Autodesk Inventor part; units mm, degrees
(part 2 of 5)
  line L843 (-13.4881, 9.0142) -> (-14.9433, 10.4694)
  line L844 (-14.9433, 10.4694) -> (-17.5891, 16.2902)
  line L845 (-17.5891, 16.2902) -> (-17.8537, 18.4068)
  line L846 (-17.8537, 18.4068) -> (-18.2506, 18.6714)
  line L847 (-18.2506, 18.6714) -> (-18.6474, 18.4068)
  line L848 (-18.6474, 18.4068) -> (-20.2349, 15.4964)
  line L849 (-20.2349, 15.4964) -> (-21.5972, 16.8588)
  line L850 (-21.5972, 16.8588) -> (-22.7485, 18.4068)
  line L851 (-22.7485, 18.4068) -> (-22.1661, 18.9123)
  line L852 (-22.1661, 18.9123) -> (-21.4256, 19.2006)
  line L853 (-21.4256, 19.2006) -> (-21.2443, 19.7141)
  line L854 (-21.2443, 19.7141) -> (-21.272, 20.1719)
  line L855 (-21.272, 20.1719) -> (-21.5088, 20.574)
  line L856 (-21.5088, 20.574) -> (-21.9547, 20.9204)
  line L857 (-21.9547, 20.9204) -> (-23.5422, 21.185)
  line L858 (-23.5422, 21.185) -> (-24.1862, 22.076)
  line L859 (-24.1862, 22.076) -> (-25.1297, 22.6402)
  line L860 (-25.1297, 22.6402) -> (-25.5266, 22.3756)
  line L861 (-25.5266, 22.3756) -> (-25.6924, 21.3319)
  line L862 (-25.6924, 21.3319) -> (-25.5933, 20.3666)
  line L863 (-25.5933, 20.3666) -> (-25.2294, 19.4798)
  line L864 (-25.2294, 19.4798) -> (-24.6006, 18.6714)
  line L865 (-24.6006, 18.6714) -> (-25.1274, 18.1853)
  line L866 (-25.1274, 18.1853) -> (-25.7912, 17.8777)
  line L867 (-25.7912, 17.8777) -> (-25.8733, 14.9576)
  line L868 (-25.8733, 14.9576) -> (-25.5266, 12.0569)
  line L869 (-25.5266, 12.0569) -> (-25.1297, 11.3954)
  line L870 (-25.1297, 11.3954) -> (-22.4839, 10.6017)
  line L871 (-22.4839, 10.6017) -> (-22.2193, 10.2048)
  line L872 (-22.2193, 10.2048) -> (-23.1911, 9.3675)
  line L873 (-23.1911, 9.3675) -> (-24.336, 8.7496)
  line L874 (-24.336, 8.7496) -> (-24.8943, 8.0539)
  line L875 (-24.8943, 8.0539) -> (-25.3009, 7.2928)
  line L876 (-25.3009, 7.2928) -> (-25.5558, 6.4664)
  line L877 (-25.5558, 6.4664) -> (-25.6589, 5.5746)
  line L878 (-25.6589, 5.5746) -> (-25.262, 5.0454)
  line L879 (-25.262, 5.0454) -> (-24.7328, 4.6485)
  line L880 (-24.7328, 4.6485) -> (-24.6006, 3.7225)
  line L881 (-24.6006, 3.7225) -> (-25.1762, 1.909)
  line L882 (-25.1762, 1.909) -> (-25.9235, 0.1506)
  line L883 (-25.9235, 0.1506) -> (-25.4768, -0.9551)
  line L884 (-25.4768, -0.9551) -> (-24.8651, -1.966)
  line L885 (-24.8651, -1.966) -> (-30.4214, -1.966)
  line L886 (-30.4214, -1.966) -> (-30.7853, -1.0092)
  line L887 (-30.7853, -1.0092) -> (-31.4797, -0.2463)
  line L888 (-31.4797, -0.2463) -> (-34.1255, -0.2463)
  line L889 (-34.1255, -0.2463) -> (-36.1099, 1.4735)
  line L890 (-36.1099, 1.4735) -> (-36.2243, 2.2225)
  line L891 (-36.2243, 2.2225) -> (-35.9776, 2.9287)
  line L892 (-35.9776, 2.9287) -> (-34.1565, 3.5577)
  line L893 (-34.1565, 3.5577) -> (-32.2735, 3.9871)
  line L894 (-32.2735, 3.9871) -> (-31.612, 4.6485)
  line L895 (-31.612, 4.6485) -> (-30.8183, 9.6756)
  line L896 (-30.8183, 9.6756) -> (-29.4953, 12.0569)
  line L897 (-29.4953, 12.0569) -> (-28.8807, 12.6734)
  line L898 (-28.8807, 12.6734) -> (-28.0401, 12.8506)
  line L899 (-28.0401, 12.8506) -> (-28.0306, 12.165)
  line L900 (-28.0306, 12.165) -> (-27.7756, 11.5277)
  line L901 (-27.7756, 11.5277) -> (-27.511, 11.66)
  line L902 (-27.511, 11.66) -> (-27.2464, 13.2475)
  line L903 (-27.2464, 13.2475) -> (-28.3047, 20.3912)
  line L904 (-28.3047, 20.3912) -> (-27.511, 22.6402)
  line L905 (-27.511, 22.6402) -> (-27.8275, 23.4912)
  line L906 (-27.8275, 23.4912) -> (-27.889, 24.3261)
  line L907 (-27.889, 24.3261) -> (-27.6953, 25.1448)
  line L908 (-27.6953, 25.1448) -> (-27.2464, 25.9475)
  line L909 (-27.2464, 25.9475) -> (-25.1306, 26.2504)
  line L910 (-25.1306, 26.2504) -> (-23.0131, 26.0798)
  line L911 (-23.0131, 26.0798) -> (-21.5599, 26.1286)
  line L912 (-21.5599, 26.1286) -> (-20.2818, 26.5197)
  line L913 (-20.2818, 26.5197) -> (-19.1787, 27.2531)
  line L914 (-19.1787, 27.2531) -> (-18.2506, 28.3287)
  line L915 (-18.2506, 28.3287) -> (-19.5551, 30.806)
  line L916 (-19.5551, 30.806) -> (-21.161, 33.0912)
  line L917 (-21.161, 33.0912) -> (-24.5793, 35.33)
  line L918 (-24.5793, 35.33) -> (-28.3047, 37.06)
  line L919 (-28.3047, 37.06) -> (-28.5692, 37.3245)
  line L920 (-28.5692, 37.3245) -> (-28.3047, 37.5891)
  line L921 (-28.3047, 37.5891) -> (-26.8515, 37.5331)
  line L922 (-26.8515, 37.5331) -> (-25.3943, 37.3245)
  line L923 (-25.3943, 37.3245) -> (-20.8964, 36.0016)
  line L924 (-20.8964, 36.0016) -> (-17.0599, 31.636)
  line L925 (-17.0599, 31.636) -> (-16.8535, 30.8052)
  line L926 (-16.8535, 30.8052) -> (-16.4539, 30.1534)
  line L927 (-16.4539, 30.1534) -> (-15.8613, 29.6807)
  line L928 (-15.8613, 29.6807) -> (-15.0756, 29.387)
  line L929 (-15.0756, 29.387) -> (-14.0172, 27.6673)
  line L930 (-14.0172, 27.6673) -> (-13.6204, 27.2703)
  line L931 (-13.6204, 27.2703) -> (-13.2235, 27.138)
  line L932 (-13.2235, 27.138) -> (-12.8266, 27.2703)
  line L933 (-12.8266, 27.2703) -> (-12.4297, 27.6673)
  line L934 (-12.4297, 27.6673) -> (-12.18, 28.5967)
  line L935 (-12.18, 28.5967) -> (-11.6999, 29.1931)
  line L936 (-11.6999, 29.1931) -> (-10.9894, 29.4565)
  line L937 (-10.9894, 29.4565) -> (-10.0485, 29.387)
  line L938 (-10.0485, 29.387) -> (-10.0048, 27.4854)
  line L939 (-10.0048, 27.4854) -> (-9.6516, 25.5506)
  line L940 (-9.6516, 25.5506) -> (-9.1787, 24.6043)
  line L941 (-9.1787, 24.6043) -> (-8.461, 23.8308)
  line L942 (-8.461, 23.8308) -> (-7.8498, 23.3711)
  line L943 (-7.8498, 23.3711) -> (-7.2491, 23.2178)
  line L944 (-7.2491, 23.2178) -> (-6.6591, 23.3711)
  line L945 (-6.6591, 23.3711) -> (-6.0797, 23.8308)
  line L946 (-6.0797, 23.8308) -> (-3.1693, 23.9631)
  line L947 (-3.1693, 23.9631) -> (-2.9048, 24.4923)
  line L948 (-2.9048, 24.4923) -> (-3.1693, 25.0214)
  line L949 (-3.1693, 25.0214) -> (-2.4802, 26.1616)
  line L950 (-2.4802, 26.1616) -> (-1.9787, 27.4027)
  line L951 (-1.9787, 27.4027) -> (-0.1266, 27.6673)
  line L952 (-0.1266, 27.6673) -> (0.0057, 28.461)
  line L953 (0.0057, 28.461) -> (-0.1266, 29.2548)
  line L954 (-0.1266, 29.2548) -> (-1.7141, 30.0485)
  line L955 (-1.7141, 30.0485) -> (-1.4495, 32.9589)
  line L956 (-1.4495, 32.9589) -> (-1.7141, 33.2235)
  line L957 (-1.7141, 33.2235) -> (-2.261, 32.8104)
  line L958 (-2.261, 32.8104) -> (-2.7299, 32.7389)
  line L959 (-2.7299, 32.7389) -> (-3.1209, 33.0089)
  line L960 (-3.1209, 33.0089) -> (-3.4339, 33.6204)
  line L961 (-3.4339, 33.6204) -> (-3.0725, 34.0812)
  line L962 (-3.0725, 34.0812) -> (-2.6654, 34.2568)
  line L963 (-2.6654, 34.2568) -> (-2.2126, 34.1473)
  line L964 (-2.2126, 34.1473) -> (-1.7141, 33.7527)
  line L965 (-1.7141, 33.7527) -> (-2.0611, 35.7499)
  line L966 (-2.0611, 35.7499) -> (-2.6402, 37.7214)
  line L967 (-2.6402, 37.7214) -> (-4.2277, 38.7797)
  line L968 (-4.2277, 38.7797) -> (-4.2715, 38.0841)
  line L969 (-4.2715, 38.0841) -> (-4.4922, 37.3245)
  line L970 (-4.4922, 37.3245) -> (-5.3543, 36.8938)
  line L971 (-5.3543, 36.8938) -> (-6.0797, 36.2662)
  line L972 (-6.0797, 36.2662) -> (-6.6089, 36.1338)
  line L973 (-6.6089, 36.1338) -> (-7.1381, 36.2662)
  line L974 (-7.1381, 36.2662) -> (-7.3598, 36.574)
  line L975 (-7.3598, 36.574) -> (-7.2704, 36.9277)
  line L976 (-7.2704, 36.9277) -> (-6.457, 37.4644)
  line L977 (-6.457, 37.4644) -> (-5.5506, 37.8537)
  line L978 (-5.5506, 37.8537) -> (-5.2207, 38.2072)
  line L979 (-5.2207, 38.2072) -> (-5.0887, 38.5675)
  line L980 (-5.0887, 38.5675) -> (-5.1545, 38.9347)
  line L981 (-5.1545, 38.9347) -> (-5.4183, 39.3089)
  line L982 (-5.4183, 39.3089) -> (-6.2965, 39.6923)
  line L983 (-6.2965, 39.6923) -> (-7.1846, 39.8201)
  line L984 (-7.1846, 39.8201) -> (-8.0825, 39.6923)
  line L985 (-8.0825, 39.6923) -> (-8.9902, 39.3089)
  line L986 (-8.9902, 39.3089) -> (-10.3341, 40.2553)
  line L987 (-10.3341, 40.2553) -> (-11.5037, 41.4256)
  line L988 (-11.5037, 41.4256) -> (-11.6909, 42.2371)
  line L989 (-11.6909, 42.2371) -> (-11.6431, 43.0148)
  line L990 (-11.6431, 43.0148) -> (-11.3602, 43.7585)
  line L991 (-11.3602, 43.7585) -> (-10.8422, 44.4683)
  line L992 (-10.8422, 44.4683) -> (-9.1611, 44.8525)
  line L993 (-9.1611, 44.8525) -> (-7.535, 45.3943)
  line L994 (-7.535, 45.3943) -> (-7.0058, 47.7756)
  line L995 (-7.0058, 47.7756) -> (-4.0954, 50.1568)
  line L996 (-4.0954, 50.1568) -> (-3.3016, 51.7443)
  line L997 (-3.3016, 51.7443) -> (-3.3753, 54.0825)
  line L998 (-3.3753, 54.0825) -> (-3.5983, 56.4054)
  line L999 (-3.5983, 56.4054) -> (-4.4922, 61.0047)
  line L1000 (-4.4922, 61.0047) -> (-4.1521, 61.7435)
  line L1001 (-4.1521, 61.7435) -> (-3.5662, 62.3276)
  line L1002 (-3.5662, 62.3276) -> (-3.1693, 63.7828)
  line L1003 (-3.1693, 63.7828) -> (-6.3443, 71.588)
  line L1004 (-6.3443, 71.588) -> (-6.0798, 72.9109)
  line L1005 (-6.0798, 72.9109) -> (-6.3443, 74.2339)
  line L1006 (-6.3443, 74.2339) -> (-6.0348, 75.915)
  line L1007 (-6.0348, 75.915) -> (-5.5506, 77.5411)
  line L1008 (-5.5506, 77.5411) -> (-5.8915, 78.1577)
  line L1009 (-5.8915, 78.1577) -> (-6.0271, 78.782)
  line L1010 (-6.0271, 78.782) -> (-5.9576, 79.4144)
  line L1011 (-5.9576, 79.4144) -> (-5.6829, 80.0547)
  line L1012 (-5.6829, 80.0547) -> (-4.5325, 80.8011)
  line L1013 (-4.5325, 80.8011) -> (-3.7742, 81.7554)
  line L1014 (-3.7742, 81.7554) -> (-3.408, 82.9177)
  line L1015 (-3.408, 82.9177) -> (-3.4339, 84.288)
  line L1016 (-3.4339, 84.288) -> (-2.6402, 84.1557)
  line L1017 (-2.6402, 84.1557) -> (-1.785, 83.346)
  line L1018 (-1.785, 83.346) -> (-1.0324, 82.8243)
  line L1019 (-1.0324, 82.8243) -> (-0.3824, 82.5906)
  line L1020 (-0.3824, 82.5906) -> (0.1649, 82.645)
  line L1021 (0.1649, 82.645) -> (0.6097, 82.9875)
  line L1022 (0.6097, 82.9875) -> (0.9519, 83.618)
  line L1023 (0.9519, 83.618) -> (1.1916, 84.5366)
  line L1024 (1.1916, 84.5366) -> (1.3286, 85.7432)
  line L1025 (1.3286, 85.7432) -> (1.2928, 86.682)
  line L1026 (1.2928, 86.682) -> (1.1044, 87.5683)
  line L1027 (1.1044, 87.5683) -> (0.7636, 88.4018)
  line L1028 (0.7636, 88.4018) -> (0.2702, 89.1828)
  line L1029 (0.2702, 89.1828) -> (-0.6682, 89.4152)
  line L1030 (-0.6682, 89.4152) -> (-1.3173, 90.1088)
  line L1031 (-1.3173, 90.1088) -> (-0.8591, 90.8667)
  line L1032 (-0.8591, 90.8667) -> (-0.2654, 91.2958)
  line L1033 (-0.2654, 91.2958) -> (0.4638, 91.3959)
  line L1034 (0.4638, 91.3959) -> (1.3286, 91.1672)
  line L1035 (1.3286, 91.1672) -> (3.1196, 87.6571)
  line L1036 (3.1196, 87.6571) -> (4.6359, 84.0234)
  line L1037 (4.6359, 84.0234) -> (4.7682, 81.6422)
  line L1038 (4.7682, 81.6422) -> (4.6359, 79.2609)
  line L1039 (4.6359, 79.2609) -> (3.588, 77.6838)
  line L1040 (3.588, 77.6838) -> (2.1223, 76.4828)
  line L1041 (2.1223, 76.4828) -> (-2.7725, 74.2339)
  line L1042 (-2.7725, 74.2339) -> (-2.9048, 72.7787)
  line L1043 (-2.9048, 72.7787) -> (-2.7725, 71.3234)
  line L1044 (-2.7725, 71.3234) -> (-2.1409, 69.1464)
  line L1045 (-2.1409, 69.1464) -> (-1.859, 68.6021)
  line L1046 (-1.859, 68.6021) -> (-1.5997, 68.4207)
  line L1047 (-1.5997, 68.4207) -> (-1.3629, 68.6021)
  line L1048 (-1.3629, 68.6021) -> (-1.1487, 69.1464)
  line L1049 (-1.1487, 69.1464) -> (-0.7881, 71.3234)
  line L1050 (-0.7881, 71.3234) -> (0.0057, 71.3234)
  line L1051 (0.0057, 71.3234) -> (-0.1433, 69.3393)
  line L1052 (-0.1433, 69.3393) -> (-0.1266, 67.3547)
  line L1053 (-0.1266, 67.3547) -> (1.4609, 64.1797)
  line L1054 (1.4609, 64.1797) -> (8.4723, 60.3433)
  line L1055 (8.4723, 60.3433) -> (9.5248, 58.7629)
  line L1056 (9.5248, 58.7629) -> (10.8536, 57.4328)
  line L1057 (10.8536, 57.4328) -> (12.4411, 57.3005)
  line L1058 (12.4411, 57.3005) -> (14.0286, 57.4328)
  line L1059 (14.0286, 57.4328) -> (14.2984, 57.8749)
  line L1060 (14.2984, 57.8749) -> (14.631, 58.1325)
  line L1061 (14.631, 58.1325) -> (15.0261, 58.2056)
  line L1062 (15.0261, 58.2056) -> (15.4838, 58.0943)
  line L1063 (15.4838, 58.0943) -> (16.2775, 58.6235)
  line L1064 (16.2775, 58.6235) -> (16.6744, 60.3433)
  line L1065 (16.6744, 60.3433) -> (17.8565, 60.6698)
  line L1066 (17.8565, 60.6698) -> (18.9233, 61.2693)
  line L1067 (18.9233, 61.2693) -> (19.3287, 60.6557)
  line L1068 (19.3287, 60.6557) -> (19.53, 60.0102)
  line L1069 (19.53, 60.0102) -> (19.5271, 59.3328)
  line L1070 (19.5271, 59.3328) -> (19.3202, 58.6235)
  line L1071 (19.3202, 58.6235) -> (16.939, 58.2266)
  line L1072 (16.939, 58.2266) -> (16.2764, 57.0344)
  line L1073 (16.2764, 57.0344) -> (15.8806, 55.7131)
  line L1074 (15.8806, 55.7131) -> (16.4047, 54.6158)
  line L1075 (16.4047, 54.6158) -> (17.1306, 54.0295)
  line L1076 (17.1306, 54.0295) -> (18.0583, 53.9543)
  line L1077 (18.0583, 53.9543) -> (19.1879, 54.3901)
  line L1078 (19.1879, 54.3901) -> (19.4525, 53.861)
  line L1079 (19.4525, 53.861) -> (19.3469, 52.5366)
  line L1080 (19.3469, 52.5366) -> (19.0556, 51.2151)
  line L1081 (19.0556, 51.2151) -> (20.2689, 48.7465)
  line L1082 (20.2689, 48.7465) -> (21.3046, 46.1881)
  line L1083 (21.3046, 46.1881) -> (21.4369, 41.5579)
  line L1084 (21.4369, 41.5579) -> (21.2638, 40.857)
  line L1085 (21.2638, 40.857) -> (20.9077, 40.2349)
  line L1086 (20.9077, 40.2349) -> (21.7155, 38.0761)
  line L1087 (21.7155, 38.0761) -> (22.3629, 35.8693)
  line L1088 (22.3629, 35.8693) -> (23.0109, 35.22)
  line L1089 (23.0109, 35.22) -> (23.8181, 34.811)
  line L1090 (-10.3131, 90.3734) -> (-9.6954, 90.1039)
  line L1091 (-9.6954, 90.1039) -> (-9.3572, 89.7053)
  line L1092 (-9.3572, 89.7053) -> (-9.2985, 89.1778)
  line L1093 (-9.2985, 89.1778) -> (-9.5193, 88.5213)
  line L1094 (-9.5193, 88.5213) -> (-10.0169, 88.885)
  line L1095 (-10.0169, 88.885) -> (-10.3151, 89.3149)
  line L1096 (-10.3151, 89.3149) -> (-10.4138, 89.8111)
  line L1097 (-10.4138, 89.8111) -> (-10.3131, 90.3734)
  line L1098 (-2.111, 81.6422) -> (-1.6804, 81.4822)
  line L1099 (-1.6804, 81.4822) -> (-1.8464, 81.113)
  line L1100 (-1.8464, 81.113) -> (-2.0709, 81.336)
  line L1101 (-2.0709, 81.336) -> (-2.111, 81.6422)
  line L1102 (0.0057, 79.7901) -> (1.064, 79.7901)
  line L1103 (1.064, 79.7901) -> (0.9372, 79.0131)
  line L1104 (0.9372, 79.0131) -> (0.5348, 78.3349)
  line L1105 (0.5348, 78.3349) -> (-1.0602, 77.6054)
  line L1106 (-1.0602, 77.6054) -> (-2.5079, 76.6151)
  line L1107 (-2.5079, 76.6151) -> (-2.9048, 77.012)
  line L1108 (-2.9048, 77.012) -> (0.0057, 79.7901)
  line L1109 (-8.9902, 68.6776) -> (-8.587, 68.1188)
  line L1110 (-8.587, 68.1188) -> (-8.3865, 67.5356)
  line L1111 (-8.3865, 67.5356) -> (-8.3886, 66.9281)
  line L1112 (-8.3886, 66.9281) -> (-8.5933, 66.2964)
  line L1113 (-8.5933, 66.2964) -> (-9.0138, 66.8348)
  line L1114 (-9.0138, 66.8348) -> (-9.2201, 67.4112)
  line L1115 (-9.2201, 67.4112) -> (-9.2123, 68.0255)
  line L1116 (-9.2123, 68.0255) -> (-8.9902, 68.6776)
  line L1117 (6.0911, 67.8839) -> (6.9693, 67.7514)
  line L1118 (6.9693, 67.7514) -> (7.5266, 67.3765)
  line L1119 (7.5266, 67.3765) -> (7.763, 66.7592)
  line L1120 (7.763, 66.7592) -> (7.6786, 65.8995)
  line L1121 (7.6786, 65.8995) -> (8.1022, 65.2041)
  line L1122 (8.1022, 65.2041) -> (8.3757, 64.4652)
  line L1123 (8.3757, 64.4652) -> (8.4991, 63.6827)
  line L1124 (8.4991, 63.6827) -> (8.4723, 62.8568)
  line L1125 (8.4723, 62.8568) -> (6.9735, 63.2176)
  line L1126 (6.9735, 63.2176) -> (5.5698, 63.7788)
  line L1127 (5.5698, 63.7788) -> (4.2615, 64.5404)
  line L1128 (4.2615, 64.5404) -> (3.0484, 65.5026)
  line L1129 (3.0484, 65.5026) -> (2.9327, 65.9263)
  line L1130 (2.9327, 65.9263) -> (3.1807, 66.2964)
  line L1131 (3.1807, 66.2964) -> (6.0911, 67.8839)
  line L1132 (12.4411, 67.3547) -> (13.0411, 67.1077)
  line L1133 (13.0411, 67.1077) -> (13.3955, 66.7166)
  line L1134 (13.3955, 66.7166) -> (13.5042, 66.1816)
  line L1135 (13.5042, 66.1816) -> (13.3671, 65.5026)
  line L1136 (13.3671, 65.5026) -> (12.876, 65.3031)
  line L1137 (12.876, 65.3031) -> (12.5138, 65.3469)
  line L1138 (12.5138, 65.3469) -> (12.2807, 65.6339)
  line L1139 (12.2807, 65.6339) -> (12.1765, 66.1641)
  line L1140 (12.1765, 66.1641) -> (12.4411, 67.3547)
  line L1141 (15.3515, 63.1214) -> (15.9294, 63.0828)
  line L1142 (15.9294, 63.0828) -> (16.2103, 62.9376)
  line L1143 (16.2103, 62.9376) -> (16.194, 62.6859)
  line L1144 (16.194, 62.6859) -> (15.8806, 62.3276)
  line L1145 (15.8806, 62.3276) -> (15.4668, 62.6263)
  line L1146 (15.4668, 62.6263) -> (15.3515, 63.1214)
  line L1147 (23.8181, 31.9006) -> (23.8181, -1.966)
  line L1148 (23.8181, -1.966) -> (15.8806, -1.966)
  line L1149 (15.8806, -1.966) -> (15.897, -0.6281)
  line L1150 (15.897, -0.6281) -> (16.1452, 0.6798)
  line L1151 (16.1452, 0.6798) -> (15.6161, 1.7381)
  line L1152 (15.6161, 1.7381) -> (14.9676, -0.0479)
  line L1153 (14.9676, -0.0479) -> (14.8223, -1.966)
  line L1154 (14.8223, -1.966) -> (6.6202, -1.966)
  line L1155 (6.6202, -1.966) -> (7.3492, -0.3101)
  line L1156 (7.3492, -0.3101) -> (8.34, 1.209)
  line L1157 (8.34, 1.209) -> (8.5694, 2.7597)
  line L1158 (8.5694, 2.7597) -> (9.131, 4.1145)
  line L1159 (9.131, 4.1145) -> (10.0246, 5.2733)
  line L1160 (10.0246, 5.2733) -> (11.2504, 6.236)
  line L1161 (11.2504, 6.236) -> (12.0442, 14.1735)
  line L1162 (12.0442, 14.1735) -> (12.3893, 14.519)
  line L1163 (12.3893, 14.519) -> (12.8379, 14.7027)
  line L1164 (12.8379, 14.7027) -> (13.382, 14.3322)
  line L1165 (13.382, 14.3322) -> (13.894, 14.2307)
  line L1166 (13.894, 14.2307) -> (14.3741, 14.3983)
  line L1167 (14.3741, 14.3983) -> (14.8223, 14.835)
  line L1168 (14.8223, 14.835) -> (14.1321, 15.4049)
  line L1169 (14.1321, 15.4049) -> (13.2348, 15.4964)
  line L1170 (13.2348, 15.4964) -> (14.69, 19.2006)
  line L1171 (14.69, 19.2006) -> (14.8337, 20.4965)
  line L1172 (14.8337, 20.4965) -> (15.2564, 21.6561)
  line L1173 (15.2564, 21.6561) -> (15.9581, 22.6793)
  line L1174 (15.9581, 22.6793) -> (16.939, 23.5662)
  line L1175 (16.939, 23.5662) -> (17.4681, 23.6986)
  line L1176 (17.4681, 23.6986) -> (17.9973, 23.5662)
  line L1177 (17.9973, 23.5662) -> (18.1939, 22.7246)
  line L1178 (18.1939, 22.7246) -> (18.6121, 22.1574)
  line L1179 (18.6121, 22.1574) -> (19.2521, 21.8647)
  line L1180 (19.2521, 21.8647) -> (20.114, 21.8464)
  line L1181 (20.114, 21.8464) -> (20.2463, 23.1693)
  line L1182 (20.2463, 23.1693) -> (20.9679, 23.6459)
  line L1183 (20.9679, 23.6459) -> (21.3627, 24.2457)
  line L1184 (21.3627, 24.2457) -> (21.4309, 24.9688)
  line L1185 (21.4309, 24.9688) -> (21.1723, 25.8152)
  line L1186 (21.1723, 25.8152) -> (21.3562, 26.4476)
  line L1187 (21.3562, 26.4476) -> (21.7015, 27.0058)
  line L1188 (21.7015, 27.0058) -> (21.1604, 28.3645)
  line L1189 (21.1604, 28.3645) -> (20.7754, 29.7839)
  line L1190 (20.7754, 29.7839) -> (18.6588, 30.8423)
  line L1191 (18.6588, 30.8423) -> (17.4681, 34.0172)
  line L1192 (17.4681, 34.0172) -> (17.1167, 32.9452)
  line L1193 (17.1167, 32.9452) -> (16.5806, 32.4555)
  line L1194 (16.5806, 32.4555) -> (15.8599, 32.5483)
  line L1195 (15.8599, 32.5483) -> (14.9546, 33.2235)
  line L1196 (14.9546, 33.2235) -> (14.4254, 35.6047)
  line L1197 (14.4254, 35.6047) -> (13.6792, 36.6144)
  line L1198 (13.6792, 36.6144) -> (13.1025, 37.7214)
  line L1199 (13.1025, 37.7214) -> (12.4382, 38.3921)
  line L1200 (12.4382, 38.3921) -> (11.7097, 38.8803)
  line L1201 (11.7097, 38.8803) -> (10.9169, 39.1859)
  line L1202 (10.9169, 39.1859) -> (10.0598, 39.3089)
  line L1203 (10.0598, 39.3089) -> (9.7952, 39.9704)
  line L1204 (9.7952, 39.9704) -> (10.3309, 40.9062)
  line L1205 (10.3309, 40.9062) -> (10.4567, 41.9547)
  line L1206 (10.4567, 41.9547) -> (9.7952, 42.2193)
  line L1207 (9.7952, 42.2193) -> (9.1338, 41.9547)
  line L1208 (9.1338, 41.9547) -> (7.8109, 42.7485)
  line L1209 (7.8109, 42.7485) -> (7.539, 42.4625)
  line L1210 (7.539, 42.4625) -> (7.414, 42.087)
  line L1211 (7.414, 42.087) -> (8.1489, 39.2799)
  line L1212 (8.1489, 39.2799) -> (8.4723, 36.3985)
  line L1213 (8.4723, 36.3985) -> (8.3656, 34.6652)
  line L1214 (8.3656, 34.6652) -> (7.6786, 33.0912)
  line L1215 (7.6786, 33.0912) -> (8.2077, 32.4297)
  line L1216 (8.2077, 32.4297) -> (9.0611, 32.9781)
  line L1217 (9.0611, 32.9781) -> (9.6322, 33.69)
  line L1218 (9.6322, 33.69) -> (9.921, 34.5656)
  line L1219 (9.921, 34.5656) -> (9.9275, 35.6047)
  line L1220 (9.9275, 35.6047) -> (10.4678, 36.4029)
  line L1221 (10.4678, 36.4029) -> (10.9346, 36.6249)
  line L1222 (10.9346, 36.6249) -> (11.3277, 36.2706)
  line L1223 (11.3277, 36.2706) -> (11.6473, 35.3402)
  line L1224 (11.6473, 35.3402) -> (13.0243, 34.2399)
  line L1225 (13.0243, 34.2399) -> (13.9684, 32.925)
  line L1226 (13.9684, 32.925) -> (14.4795, 31.3956)
  line L1227 (14.4795, 31.3956) -> (14.5577, 29.6516)
  line L1228 (14.5577, 29.6516) -> (13.5917, 29.6284)
  line L1229 (13.5917, 29.6284) -> (12.7056, 30.0485)
  line L1230 (12.7056, 30.0485) -> (12.3088, 29.2548)
  line L1231 (12.3088, 29.2548) -> (12.3439, 26.9951)
  line L1232 (12.3439, 26.9951) -> (12.7056, 24.7568)
  line L1233 (12.7056, 24.7568) -> (12.2496, 22.1378)
  line L1234 (12.2496, 22.1378) -> (12.1765, 19.4652)
  line L1235 (12.1765, 19.4652) -> (12.7014, 19.4555)
  line L1236 (12.7014, 19.4555) -> (13.0087, 19.298)
  line L1237 (13.0087, 19.298) -> (13.0983, 18.9926)
  line L1238 (13.0983, 18.9926) -> (12.9702, 18.5391)
  line L1239 (12.9702, 18.5391) -> (12.0111, 18.2994)
  line L1240 (12.0111, 18.2994) -> (11.1181, 17.8777)
  line L1241 (11.1181, 17.8777) -> (10.7439, 18.6086)
  line L1242 (10.7439, 18.6086) -> (10.1921, 19.2006)
  line L1243 (10.1921, 19.2006) -> (8.7369, 17.4808)
  line L1244 (8.7369, 17.4808) -> (8.3833, 17.3914)
  line L1245 (8.3833, 17.3914) -> (8.0754, 17.6131)
  line L1246 (8.0754, 17.6131) -> (9.5306, 26.8735)
  line L1247 (9.5306, 26.8735) -> (8.8807, 29.2136)
  line L1248 (8.8807, 29.2136) -> (7.8109, 31.3714)
  line L1249 (7.8109, 31.3714) -> (7.0286, 30.5893)
  line L1250 (7.0286, 30.5893) -> (6.7525, 29.5193)
  line L1251 (6.7525, 29.5193) -> (6.0366, 30.7639)
  line L1252 (6.0366, 30.7639) -> (5.165, 31.9006)
  line L1253 (5.165, 31.9006) -> (4.7381, 31.4459)
  line L1254 (4.7381, 31.4459) -> (4.4636, 30.9416)
  line L1255 (4.4636, 30.9416) -> (4.3413, 30.3876)
  line L1256 (4.3413, 30.3876) -> (4.3713, 29.7839)
  line L1257 (4.3713, 29.7839) -> (4.9502, 28.0407)
  line L1258 (4.9502, 28.0407) -> (5.8265, 26.4766)
  line L1259 (5.8265, 26.4766) -> (4.7682, 23.0371)
  line L1260 (4.7682, 23.0371) -> (4.0854, 22.9998)
  line L1261 (4.0854, 22.9998) -> (3.7098, 23.5662)
  line L1262 (3.7098, 23.5662) -> (4.0622, 24.4023)
  line L1263 (4.0622, 24.4023) -> (4.239, 25.286)
  line L1264 (4.239, 25.286) -> (3.6042, 25.1314)
  line L1265 (3.6042, 25.1314) -> (3.1059, 24.8153)
  line L1266 (3.1059, 24.8153) -> (2.7443, 24.3377)
  line L1267 (2.7443, 24.3377) -> (2.5192, 23.6985)
  line L1268 (2.5192, 23.6985) -> (1.99, 24.2277)
  line L1269 (1.99, 24.2277) -> (1.064, 30.3131)
  line L1270 (1.064, 30.3131) -> (1.7255, 34.2818)
  line L1271 (1.7255, 34.2818) -> (-0.1266, 38.7797)
  line L1272 (-0.1266, 38.7797) -> (-0.96, 39.894)
  line L1273 (-0.96, 39.894) -> (-1.304, 41.0592)
  line L1274 (-1.304, 41.0592) -> (-1.1585, 42.2753)
  line L1275 (-1.1585, 42.2753) -> (-0.5235, 43.5422)
  line L1276 (-0.5235, 43.5422) -> (-1.5818, 45.262)
  line L1277 (-1.5818, 45.262) -> (-1.185, 47.7756)
  line L1278 (-1.185, 47.7756) -> (0.1388, 49.1654)
  line L1279 (0.1388, 49.1654) -> (1.5932, 50.4214)
  line L1280 (1.5932, 50.4214) -> (-0.7881, 51.3474)
  line L1281 (-0.7881, 51.3474) -> (-1.4495, 52.0089)
  line L1282 (-1.4495, 52.0089) -> (-1.9988, 54.8951)
  line L1283 (-1.9988, 54.8951) -> (-1.9787, 57.8297)
  line L1284 (-1.9787, 57.8297) -> (-0.794, 58.2255)
  line L1285 (-0.794, 58.2255) -> (0.2702, 58.888)
  line L1286 (0.2702, 58.888) -> (-0.9597, 59.0965)
  line L1287 (-0.9597, 59.0965) -> (-1.7004, 59.651)
  line L1288 (-1.7004, 59.651) -> (-1.9519, 60.5517)
  line L1289 (-1.9519, 60.5517) -> (-1.7141, 61.7985)
  line L1290 (-1.7141, 61.7985) -> (-1.5099, 62.4174)
  line L1291 (-1.5099, 62.4174) -> (-1.0527, 62.8568)
  line L1292 (-1.0527, 62.8568) -> (-0.2869, 62.2233)
  line L1293 (-0.2869, 62.2233) -> (0.2702, 61.4016)
  line L1294 (0.2702, 61.4016) -> (1.4363, 61.0117)
  line L1295 (1.4363, 61.0117) -> (2.5192, 60.4755)
  line L1296 (2.5192, 60.4755) -> (2.7802, 59.9612)
  line L1297 (2.7802, 59.9612) -> (2.7838, 59.4172)
  line L1298 (2.7838, 59.4172) -> (1.064, 58.3589)
  line L1299 (1.064, 58.3589) -> (3.1807, 56.1099)
  line L1300 (3.1807, 56.1099) -> (3.667, 56.0073)
  line L1301 (3.667, 56.0073) -> (4.1067, 56.2422)
  line L1302 (4.1067, 56.2422) -> (5.5619, 59.6818)
  line L1303 (5.5619, 59.6818) -> (6.2596, 59.0815)
  line L1304 (6.2596, 59.0815) -> (6.6202, 58.2266)
  line L1305 (6.6202, 58.2266) -> (6.2148, 57.2681)
  line L1306 (6.2148, 57.2681) -> (6.2234, 56.2422)
  line L1307 (6.2234, 56.2422) -> (7.1968, 54.474)
  line L1308 (7.1968, 54.474) -> (8.34, 52.8026)
  line L1309 (8.34, 52.8026) -> (8.8692, 50.4214)
  line L1310 (8.8692, 50.4214) -> (9.6544, 49.9011)
  line L1311 (9.6544, 49.9011) -> (10.3244, 49.2308)
  line L1312 (10.3244, 49.2308) -> (11.1249, 49.1663)
  line L1313 (11.1249, 49.1663) -> (11.7796, 49.6276)
  line L1314 (11.7796, 49.6276) -> (12.0236, 51.101)
  line L1315 (12.0236, 51.101) -> (12.7056, 52.4058)
  line L1316 (12.7056, 52.4058) -> (13.1025, 52.5381)
  line L1317 (13.1025, 52.5381) -> (13.4994, 52.4058)
  line L1318 (13.4994, 52.4058) -> (14.0409, 51.8708)
  line L1319 (14.0409, 51.8708) -> (14.69, 51.4797)
  line L1320 (14.69, 51.4797) -> (14.8224, 50.686)
  line L1321 (14.8224, 50.686) -> (14.69, 49.8922)
  line L1322 (14.69, 49.8922) -> (13.4826, 47.89)
  line L1323 (13.4826, 47.89) -> (12.4411, 45.7912)
  line L1324 (12.4411, 45.7912) -> (13.4169, 41.5405)
  line L1325 (13.4169, 41.5405) -> (14.9546, 37.4568)
  line L1326 (14.9546, 37.4568) -> (15.9392, 36.2073)
  line L1327 (15.9392, 36.2073) -> (17.0713, 35.0756)
  line L1328 (17.0713, 35.0756) -> (17.865, 38.2506)
  line L1329 (17.865, 38.2506) -> (18.9426, 36.0792)
  line L1330 (18.9426, 36.0792) -> (19.7171, 33.7527)
  line L1331 (19.7171, 33.7527) -> (20.5861, 32.9461)
  line L1332 (20.5861, 32.9461) -> (21.5594, 32.3685)
  line L1333 (21.5594, 32.3685) -> (22.6367, 32.02)
  line L1334 (22.6367, 32.02) -> (23.8181, 31.9006)
  line L1335 (-68.2568, 59.9464) -> (-67.9922, 60.211)
  line L1336 (-67.9922, 60.211) -> (-66.4047, 59.0203)
  line L1337 (-66.4047, 59.0203) -> (-66.1725, 58.5882)
  line L1338 (-66.1725, 58.5882) -> (-66.1401, 58.0943)
  line L1339 (-66.1401, 58.0943) -> (-67.1984, 58.2266)
  line L1340 (-67.1984, 58.2266) -> (-68.2568, 59.9464)
  line L1341 (-107.1505, 58.3589) -> (-104.24, 58.3589)
  line L1342 (-104.24, 58.3589) -> (-104.1851, 57.4227)
  line L1343 (-104.1851, 57.4227) -> (-103.9755, 56.5068)
  line L1344 (-103.9755, 56.5068) -> (-104.361, 55.5334)
  line L1345 (-104.361, 55.5334) -> (-104.4233, 54.5916)
  line L1346 (-104.4233, 54.5916) -> (-104.1625, 53.6814)
  line L1347 (-104.1625, 53.6814) -> (-103.5786, 52.8026)
  line L1348 (-103.5786, 52.8026) -> (-102.1234, 57.1683)
  line L1349 (-102.1234, 57.1683) -> (-101.3869, 57.1798)
  line L1350 (-101.3869, 57.1798) -> (-100.8768, 56.9411)
  line L1351 (-100.8768, 56.9411) -> (-100.5931, 56.4522)
  line L1352 (-100.5931, 56.4522) -> (-100.5359, 55.7131)
  line L1353 (-100.5359, 55.7131) -> (-100.8986, 52.3955)
  line L1354 (-100.8986, 52.3955) -> (-101.4619, 49.0985)
  line L1355 (-101.4619, 49.0985) -> (-103.1817, 48.3047)
  line L1356 (-103.1817, 48.3047) -> (-103.5786, 48.5693)
  line L1357 (-103.5786, 48.5693) -> (-103.8432, 51.2151)
  line L1358 (-103.8432, 51.2151) -> (-105.1107, 53.2211)
  line L1359 (-105.1107, 53.2211) -> (-105.9598, 55.4485)
  line L1360 (-105.9598, 55.4485) -> (-106.4132, 55.7207)
  line L1361 (-106.4132, 55.7207) -> (-106.851, 55.7453)
  line L1362 (-106.851, 55.7453) -> (-107.2731, 55.5223)
  line L1363 (-107.2731, 55.5223) -> (-107.6796, 55.0516)
  line L1364 (-107.6796, 55.0516) -> (-108.5645, 54.7459)
  line L1365 (-108.5645, 54.7459) -> (-109.058, 54.8424)
  line L1366 (-109.058, 54.8424) -> (-109.1599, 55.3412)
  line L1367 (-109.1599, 55.3412) -> (-108.8702, 56.2422)
  line L1368 (-108.8702, 56.2422) -> (-107.7753, 57.109)
  line L1369 (-107.7753, 57.109) -> (-107.1505, 58.3589)
  line L1370 (18.7911, 57.3006) -> (19.5848, 57.3006)
  line L1371 (19.5848, 57.3006) -> (19.56, 56.1966)
  line L1372 (19.56, 56.1966) -> (19.1879, 55.1839)
  line L1373 (19.1879, 55.1839) -> (18.5677, 55.6144)
  line L1374 (18.5677, 55.6144) -> (18.2948, 56.1108)
  line L1375 (18.2948, 56.1108) -> (18.3692, 56.6728)
  line L1376 (18.3692, 56.6728) -> (18.7911, 57.3006)
  line L1377 (-116.1463, 54.1256) -> (-115.3293, 54.2375)
  line L1378 (-115.3293, 54.2375) -> (-114.5278, 54.1646)
  line L1379 (-114.5278, 54.1646) -> (-113.7418, 53.9068)
  line L1380 (-113.7418, 53.9068) -> (-112.9713, 53.4641)
  line L1381 (-112.9713, 53.4641) -> (-110.0609, 53.1995)
  line L1382 (-110.0609, 53.1995) -> (-109.0025, 52.4058)
  line L1383 (-109.0025, 52.4058) -> (-109.7988, 51.8387)
  line L1384 (-109.7988, 51.8387) -> (-110.6375, 51.5615)
  line L1385 (-110.6375, 51.5615) -> (-111.5186, 51.5742)
  line L1386 (-111.5186, 51.5742) -> (-112.4421, 51.8766)
  line L1387 (-112.4421, 51.8766) -> (-116.1463, 54.1256)
  line L1388 (-107.6796, 53.861) -> (-107.2185, 53.6233)
  line L1389 (-107.2185, 53.6233) -> (-107.0207, 53.3456)
  line L1390 (-107.0207, 53.3456) -> (-107.0862, 53.028)
  line L1391 (-107.0862, 53.028) -> (-107.415, 52.6703)
  line L1392 (-107.415, 52.6703) -> (-108.0765, 52.538)
  line L1393 (-108.0765, 52.538) -> (-108.738, 52.6703)
  line L1394 (-108.738, 52.6703) -> (-107.6796, 53.861)
  line L1395 (-12.9589, 53.5964) -> (-12.1652, 53.5964)
  line L1396 (-12.1652, 53.5964) -> (-12.4781, 52.6182)
  line L1397 (-12.4781, 52.6182) -> (-13.2235, 51.8766)
  line L1398 (-13.2235, 51.8766) -> (-14.4246, 51.3256)
  line L1399 (-14.4246, 51.3256) -> (-15.377, 50.6769)
  line L1400 (-15.377, 50.6769) -> (-16.0808, 49.9305)
  line L1401 (-16.0808, 49.9305) -> (-16.5358, 49.0864)
  line L1402 (-16.5358, 49.0864) -> (-16.7422, 48.1446)
  line L1403 (-16.7422, 48.1446) -> (-16.6999, 47.105)
  line L1404 (-16.6999, 47.105) -> (-16.409, 45.9678)
  line L1405 (-16.409, 45.9678) -> (-15.8693, 44.7329)
  line L1406 (-15.8693, 44.7329) -> (-16.782, 43.2532)
  line L1407 (-16.782, 43.2532) -> (-17.1507, 42.9246)
  line L1408 (-17.1507, 42.9246) -> (-17.461, 42.8703)
  line L1409 (-17.461, 42.8703) -> (-17.7129, 43.09)
  line L1410 (-17.7129, 43.09) -> (-17.9064, 43.584)
  line L1411 (-17.9064, 43.584) -> (-18.1183, 45.3943)
  line L1412 (-18.1183, 45.3943) -> (-18.5178, 46.0583)
  line L1413 (-18.5178, 46.0583) -> (-19.1766, 46.4526)
  line L1414 (-19.1766, 46.4526) -> (-20.9302, 45.7744)
  line L1415 (-20.9302, 45.7744) -> (-22.4839, 44.7329)
  line L1416 (-22.4839, 44.7329) -> (-23.3922, 44.4539)
  line L1417 (-23.3922, 44.4539) -> (-24.336, 44.336)
  line L1418 (-24.336, 44.336) -> (-27.511, 45.262)
  line L1419 (-27.511, 45.262) -> (-27.8846, 45.7271)
  line L1420 (-27.8846, 45.7271) -> (-27.943, 46.1247)
  line L1421 (-27.943, 46.1247) -> (-27.6861, 46.4547)
  line L1422 (-27.6861, 46.4547) -> (-27.1141, 46.7172)
  line L1423 (-27.1141, 46.7172) -> (-26.4475, 46.1841)
  line L1424 (-26.4475, 46.1841) -> (-26.0558, 45.3943)
  line L1425 (-26.0558, 45.3943) -> (-25.4494, 46.0017)
  line L1426 (-25.4494, 46.0017) -> (-24.7328, 46.4526)
  line L1427 (-24.7328, 46.4526) -> (-23.983, 46.2228)
  line L1428 (-23.983, 46.2228) -> (-23.3581, 46.3005)
  line L1429 (-23.3581, 46.3005) -> (-22.8584, 46.6858)
  line L1430 (-22.8584, 46.6858) -> (-22.4839, 47.3787)
  line L1431 (-22.4839, 47.3787) -> (-21.3502, 47.4813)
  line L1432 (-21.3502, 47.4813) -> (-20.2349, 47.2464)
  line L1433 (-20.2349, 47.2464) -> (-19.4047, 47.5601)
  line L1434 (-19.4047, 47.5601) -> (-18.9074, 48.0616)
  line L1435 (-18.9074, 48.0616) -> (-18.7432, 48.7507)
  line L1436 (-18.7432, 48.7507) -> (-18.912, 49.6276)
  line L1437 (-18.912, 49.6276) -> (-20.0407, 50.2869)
  line L1438 (-20.0407, 50.2869) -> (-20.3642, 50.6584)
  line L1439 (-20.3642, 50.6584) -> (-20.5271, 51.0578)
  line L1440 (-20.5271, 51.0578) -> (-20.5295, 51.4852)
  line L1441 (-20.5295, 51.4852) -> (-20.3714, 51.9405)
  line L1442 (-20.3714, 51.9405) -> (-19.5735, 52.9349)
  line L1443 (-19.5735, 52.9349) -> (-18.9969, 53.0233)
  line L1444 (-18.9969, 53.0233) -> (-18.496, 52.9204)
  line L1445 (-18.496, 52.9204) -> (-18.0708, 52.6264)
  line L1446 (-18.0708, 52.6264) -> (-17.7214, 52.1412)
  line L1447 (-17.7214, 52.1412) -> (-16.6631, 52.0088)
  line L1448 (-16.6631, 52.0088) -> (-15.6047, 52.1412)
  line L1449 (-15.6047, 52.1412) -> (-12.9589, 53.5964)
  line L1450 (-71.6963, 52.2735) -> (-71.0548, 51.9656)
  line L1451 (-71.0548, 51.9656) -> (-70.6645, 51.5323)
  line L1452 (-70.6645, 51.5323) -> (-70.5256, 50.9735)
  line L1453 (-70.5256, 50.9735) -> (-70.638, 50.2891)
  line L1454 (-70.638, 50.2891) -> (-71.1243, 50.1865)
  line L1455 (-71.1243, 50.1865) -> (-71.564, 50.4214)
  line L1456 (-71.564, 50.4214) -> (-71.8779, 51.3494)
  line L1457 (-71.8779, 51.3494) -> (-71.6963, 52.2735)
  line L1458 (-88.1005, -1.966) -> (-91.5401, -1.966)
  line L1459 (-91.5401, -1.966) -> (-91.9757, 0.2264)
  line L1460 (-91.9757, 0.2264) -> (-92.863, 2.2673)
  line L1461 (-92.863, 2.2673) -> (-93.4772, 1.7841)
  line L1462 (-93.4772, 1.7841) -> (-94.1859, 1.4735)
  line L1463 (-94.1859, 1.4735) -> (-94.7538, 1.9282)
  line L1464 (-94.7538, 1.9282) -> (-95.1856, 2.4766)
  line L1465 (-95.1856, 2.4766) -> (-95.4814, 3.1188)
  line L1466 (-95.4814, 3.1188) -> (-95.6411, 3.8548)
  line L1467 (-95.6411, 3.8548) -> (-96.3265, 4.2758)
  line L1468 (-96.3265, 4.2758) -> (-96.8637, 4.813)
  line L1469 (-96.8637, 4.813) -> (-97.2526, 5.4664)
  line L1470 (-97.2526, 5.4664) -> (-97.4932, 6.236)
  line L1471 (-97.4932, 6.236) -> (-98.1546, 6.7652)
  line L1472 (-98.1546, 6.7652) -> (-100.2713, 5.9714)
  line L1473 (-100.2713, 5.9714) -> (-100.6806, 5.3724)
  line L1474 (-100.6806, 5.3724) -> (-100.8005, 4.6485)
  line L1475 (-100.8005, 4.6485) -> (-100.139, 1.209)
  line L1476 (-100.139, 1.209) -> (-99.3742, -0.3196)
  line L1477 (-99.3742, -0.3196) -> (-98.9484, -1.966)
  line L1478 (-98.9484, -1.966) -> (-109.2671, -1.966)
  line L1479 (-109.2671, -1.966) -> (-108.4734, -0.114)
  line L1480 (-108.4734, -0.114) -> (-109.664, 1.4735)
  line L1481 (-109.664, 1.4735) -> (-109.5755, 2.8028)
  line L1482 (-109.5755, 2.8028) -> (-109.2671, 4.1194)
  line L1483 (-109.2671, 4.1194) -> (-109.34, 4.708)
  line L1484 (-109.34, 4.708) -> (-109.5628, 5.0806)
  line L1485 (-109.5628, 5.0806) -> (-109.9354, 5.2372)
  line L1486 (-109.9354, 5.2372) -> (-110.4577, 5.1777)
  line L1487 (-110.4577, 5.1777) -> (-110.4665, 1.5949)
  line L1488 (-110.4665, 1.5949) -> (-110.0609, -1.966)
  line L1489 (-110.0609, -1.966) -> (-111.6484, -1.966)
  line L1490 (-111.6484, -1.966) -> (-111.6479, 0.2321)
  line L1491 (-111.6479, 0.2321) -> (-111.802, 2.42)
  line L1492 (-111.802, 2.42) -> (-112.1109, 4.5977)
  line L1493 (-112.1109, 4.5977) -> (-112.5744, 6.7652)
  line L1494 (-112.5744, 6.7652) -> (-113.3653, 7.6773)
  line L1495 (-113.3653, 7.6773) -> (-113.6327, 8.8819)
  line L1496 (-113.6327, 8.8819) -> (-114.4461, 9.4186)
  line L1497 (-114.4461, 9.4186) -> (-115.3525, 9.8079)
  line L1498 (-115.3525, 9.8079) -> (-116.4109, 11.3954)
  line L1499 (-116.4109, 11.3954) -> (-117.2046, 11.5277)
  line L1500 (-117.2046, 11.5277) -> (-116.4749, 9.612)
  line L1501 (-116.4749, 9.612) -> (-116.014, 7.5589)
  line L1502 (-116.014, 7.5589) -> (-115.2202, 6.236)
  line L1503 (-115.2202, 6.236) -> (-115.0879, 1.4735)
  line L1504 (-115.0879, 1.4735) -> (-115.6171, 0.1506)
  line L1505 (-115.6171, 0.1506) -> (-115.0879, -1.966)
  line L1506 (-115.0879, -1.966) -> (-118.2629, -1.966)
  line L1507 (-118.2629, -1.966) -> (-118.2995, -0.9578)
  line L1508 (-118.2995, -0.9578) -> (-118.488, -0.0044)
  line L1509 (-118.488, -0.0044) -> (-118.8286, 0.8942)
  line L1510 (-118.8286, 0.8942) -> (-119.3213, 1.7381)
  line L1511 (-119.3213, 1.7381) -> (-120.0077, 0.6128)
  line L1512 (-120.0077, 0.6128) -> (-120.5119, -0.6431)
  line L1513 (-120.5119, -0.6431) -> (-121.7025, -1.966)
  line L1514 (-121.7025, -1.966) -> (-121.9671, -1.966)
  line L1515 (-121.9671, -1.966) -> (-122.1113, -1.2417)
  line L1516 (-122.1113, -1.2417) -> (-122.4019, -0.6034)
  line L1517 (-122.4019, -0.6034) -> (-122.8389, -0.0511)
  line L1518 (-122.8389, -0.0511) -> (-123.4223, 0.4152)
  line L1519 (-123.4223, 0.4152) -> (-123.3892, 1.4194)
  line L1520 (-123.3892, 1.4194) -> (-123.6207, 2.3274)
  line L1521 (-123.6207, 2.3274) -> (-124.1168, 3.1392)
  line L1522 (-124.1168, 3.1392) -> (-124.8775, 3.8548)
  line L1523 (-124.8775, 3.8548) -> (-123.7389, 6.5591)
  line L1524 (-123.7389, 6.5591) -> (-122.364, 9.1464)
  line L1525 (-122.364, 9.1464) -> (-121.7025, 10.8662)
  line L1526 (-121.7025, 10.8662) -> (-122.4992, 11.6625)
  line L1527 (-122.4992, 11.6625) -> (-123.4223, 12.3214)
  line L1528 (-123.4223, 12.3214) -> (-124.0107, 11.6508)
  line L1529 (-124.0107, 11.6508) -> (-124.4273, 10.898)
  line L1530 (-124.4273, 10.898) -> (-124.6722, 10.0633)
  line L1531 (-124.6722, 10.0633) -> (-124.7452, 9.1464)
  line L1532 (-124.7452, 9.1464) -> (-125.3904, 8.6775)
  line L1533 (-125.3904, 8.6775) -> (-126.2004, 8.7496)
  line L1534 (-126.2004, 8.7496) -> (-127.7175, 10.2672)
  line L1535 (-127.7175, 10.2672) -> (-129.1108, 11.9246)
  line L1536 (-129.1108, 11.9246) -> (-129.3754, 12.0569)
  line L1537 (-129.3754, 12.0569) -> (-129.64, 11.9246)
  line L1538 (-129.64, 11.9246) -> (-130.3757, 8.9224)
  line L1539 (-130.3757, 8.9224) -> (-131.3598, 5.9714)
  line L1540 (-131.3598, 5.9714) -> (-131.8823, 5.5327)
  line L1541 (-131.8823, 5.5327) -> (-132.5504, 5.5746)
  line L1542 (-132.5504, 5.5746) -> (-134.1379, 8.3527)
  line L1543 (-134.1379, 8.3527) -> (-133.9751, 8.9632)
  line L1544 (-133.9751, 8.9632) -> (-133.6783, 9.4754)
  line L1545 (-133.6783, 9.4754) -> (-133.2475, 9.8893)
  line L1546 (-133.2475, 9.8893) -> (-132.6827, 10.2048)
  line L1547 (-132.6827, 10.2048) -> (-132.3921, 12.5803)
  line L1548 (-132.3921, 12.5803) -> (-132.4181, 14.9673)
  line L1549 (-132.4181, 14.9673) -> (-134.0308, 16.6044)
  line L1550 (-134.0308, 16.6044) -> (-135.4608, 18.4068)
  line L1551 (-135.4608, 18.4068) -> (-134.8785, 18.9123)
  line L1552 (-134.8785, 18.9123) -> (-134.1379, 19.2006)
  line L1553 (-134.1379, 19.2006) -> (-133.9429, 19.7415)
  line L1554 (-133.9429, 19.7415) -> (-133.9882, 20.1864)
  line L1555 (-133.9882, 20.1864) -> (-134.2737, 20.5353)
  line L1556 (-134.2737, 20.5353) -> (-134.7994, 20.7881)
  line L1557 (-134.7994, 20.7881) -> (-135.2614, 20.6188)
  line L1558 (-135.2614, 20.6188) -> (-135.7254, 20.6558)
  line L1559 (-135.7254, 20.6558) -> (-136.1751, 21.2562)
  line L1560 (-136.1751, 21.2562) -> (-136.7219, 21.6547)
  line L1561 (-136.7219, 21.6547) -> (-137.3657, 21.8515)
  line L1562 (-137.3657, 21.8515) -> (-138.1067, 21.8464)
  line L1563 (-138.1067, 21.8464) -> (-138.1067, 28.9902)
  line L1564 (-138.1067, 28.9902) -> (-137.7098, 29.5193)
  line L1565 (-137.7098, 29.5193) -> (-137.4797, 31.5928)
  line L1566 (-137.4797, 31.5928) -> (-137.0483, 33.6204)
  line L1567 (-137.0483, 33.6204) -> (-136.998, 34.2462)
  line L1568 (-136.998, 34.2462) -> (-137.1575, 34.6973)
  line L1569 (-137.1575, 34.6973) -> (-137.5271, 34.9738)
  line L1570 (-137.5271, 34.9738) -> (-138.1067, 35.0756)
  line L1571 (-138.1067, 35.0756) -> (-138.1067, 37.1922)
  line L1572 (-138.1067, 37.1922) -> (-137.3118, 37.3991)
  line L1573 (-137.3118, 37.3991) -> (-136.8484, 37.7767)
  line L1574 (-136.8484, 37.7767) -> (-136.7165, 38.3251)
  line L1575 (-136.7165, 38.3251) -> (-136.916, 39.0443)
  line L1576 (-136.916, 39.0443) -> (-138.1067, 38.5152)
  line L1577 (-138.1067, 38.5152) -> (-138.1067, 42.4839)
  line L1578 (-138.1067, 42.4839) -> (-137.6691, 42.2714)
  line L1579 (-137.6691, 42.2714) -> (-137.2587, 42.2446)
  line L1580 (-137.2587, 42.2446) -> (-136.8754, 42.4036)
  line L1581 (-136.8754, 42.4036) -> (-136.5192, 42.7485)
  line L1582 (-136.5192, 42.7485) -> (-135.7239, 44.1398)
  line L1583 (-135.7239, 44.1398) -> (-135.3486, 45.5738)
  line L1584 (-135.3486, 45.5738) -> (-135.3932, 47.0503)
  line L1585 (-135.3932, 47.0503) -> (-135.8577, 48.5693)
  line L1586 (-135.8577, 48.5693) -> (-136.9146, 49.1321)
  line L1587 (-136.9146, 49.1321) -> (-138.1067, 49.3631)
  line L1588 (-138.1067, 49.3631) -> (-138.1067, 50.686)
  line L1589 (-138.1067, 50.686) -> (-135.99, 51.4797)
  line L1590 (-135.99, 51.4797) -> (-134.113, 48.7901)
  line L1591 (-134.113, 48.7901) -> (-132.4181, 45.9235)
  line L1592 (-132.4181, 45.9235) -> (-131.889, 43.8068)
  line L1593 (-131.889, 43.8068) -> (-131.7567, 39.9704)
  line L1594 (-131.7567, 39.9704) -> (-132.2984, 38.7322)
  line L1595 (-132.2984, 38.7322) -> (-133.0302, 37.636)
  line L1596 (-133.0302, 37.636) -> (-133.952, 36.6817)
  line L1597 (-133.952, 36.6817) -> (-135.064, 35.8693)
  line L1598 (-135.064, 35.8693) -> (-135.7254, 33.6204)
  line L1599 (-135.7254, 33.6204) -> (-134.7994, 27.1381)
  line L1600 (-134.7994, 27.1381) -> (-134.1379, 26.6089)
  line L1601 (-134.1379, 26.6089) -> (-132.5504, 28.0641)
  line L1602 (-132.5504, 28.0641) -> (-130.8682, 28.2741)
  line L1603 (-130.8682, 28.2741) -> (-129.2431, 28.7256)
  line L1604 (-129.2431, 28.7256) -> (-127.9352, 28.4335)
  line L1605 (-127.9352, 28.4335) -> (-126.8619, 27.6673)
  line L1606 (-126.8619, 27.6673) -> (-126.8503, 28.4975)
  line L1607 (-126.8503, 28.4975) -> (-126.3327, 29.2548)
  line L1608 (-126.3327, 29.2548) -> (-125.4067, 28.1964)
  line L1609 (-125.4067, 28.1964) -> (-124.935, 28.9483)
  line L1610 (-124.935, 28.9483) -> (-124.6129, 29.7839)
  line L1611 (-124.6129, 29.7839) -> (-122.7609, 30.1808)
  line L1612 (-122.7609, 30.1808) -> (-121.2131, 32.8805)
  line L1613 (-121.2131, 32.8805) -> (-119.3213, 35.3402)
  line L1614 (-119.3213, 35.3402) -> (-118.1306, 39.0443)
  line L1615 (-118.1306, 39.0443) -> (-116.3447, 41.0948)
  line L1616 (-116.3447, 41.0948) -> (-114.2942, 42.8808)
  line L1617 (-114.2942, 42.8808) -> (-106.8859, 45.1297)
  line L1618 (-106.8859, 45.1297) -> (-106.7021, 46.349)
  line L1619 (-106.7021, 46.349) -> (-106.3322, 46.8657)
  line L1620 (-106.3322, 46.8657) -> (-106.0774, 46.8605)
  line L1621 (-106.0774, 46.8605) -> (-105.7761, 46.6797)
  line L1622 (-105.7761, 46.6797) -> (-105.0338, 45.7912)
  line L1623 (-105.0338, 45.7912) -> (-103.4463, 44.8651)
  line L1624 (-103.4463, 44.8651) -> (-103.2606, 44.522)
  line L1625 (-103.2606, 44.522) -> (-103.2428, 44.2091)
  line L1626 (-103.2428, 44.2091) -> (-103.7109, 43.6745)
  line L1627 (-103.7109, 43.6745) -> (-105.6681, 43.9796)
  line L1628 (-105.6681, 43.9796) -> (-107.6796, 43.9391)
  line L1629 (-107.6796, 43.9391) -> (-110.9751, 42.424)
  line L1630 (-110.9751, 42.424) -> (-114.0296, 40.4995)
  line L1631 (-114.0296, 40.4995) -> (-118.9244, 32.9589)
  line L1632 (-118.9244, 32.9589) -> (-120.4424, 29.6571)
  line L1633 (-120.4424, 29.6571) -> (-122.364, 26.6089)
  line L1634 (-122.364, 26.6089) -> (-122.3777, 25.4651)
  line L1635 (-122.3777, 25.4651) -> (-122.0074, 24.6649)
  line L1636 (-122.0074, 24.6649) -> (-121.2532, 24.2083)
  line L1637 (-121.2532, 24.2083) -> (-120.115, 24.0954)
  line L1638 (-120.115, 24.0954) -> (-118.8833, 25.3751)
  line L1639 (-118.8833, 25.3751) -> (-117.4692, 26.4766)
  line L1640 (-117.4692, 26.4766) -> (-112.7666, 28.8275)
  line L1641 (-112.7666, 28.8275) -> (-108.3411, 31.636)
  line L1642 (-108.3411, 31.636) -> (-106.8859, 30.8423)
  line L1643 (-106.8859, 30.8423) -> (-105.957, 30.9799)
  line L1644 (-105.957, 30.9799) -> (-105.5593, 30.8274)
  line L1645 (-105.5593, 30.8274) -> (-105.6925, 30.3846)
  line L1646 (-105.6925, 30.3846) -> (-106.3567, 29.6516)
  line L1647 (-106.3567, 29.6516) -> (-107.9069, 29.4233)
  line L1648 (-107.9069, 29.4233) -> (-109.3055, 28.9063)
  line L1649 (-109.3055, 28.9063) -> (-110.5527, 28.1004)
  line L1650 (-110.5527, 28.1004) -> (-111.6484, 27.0058)
  line L1651 (-111.6484, 27.0058) -> (-114.266, 26.1329)
  line L1652 (-114.266, 26.1329) -> (-116.8077, 25.0214)
  line L1653 (-116.8077, 25.0214) -> (-116.807, 24.0539)
  line L1654 (-116.807, 24.0539) -> (-116.5643, 23.1802)
  line L1655 (-116.5643, 23.1802) -> (-116.0794, 22.4002)
  line L1656 (-116.0794, 22.4002) -> (-115.3525, 21.7141)
  line L1657 (-115.3525, 21.7141) -> (-114.9557, 21.5818)
  line L1658 (-114.9557, 21.5818) -> (-114.5588, 21.7141)
  line L1659 (-114.5588, 21.7141) -> (-113.7529, 22.5242)
  line L1660 (-113.7529, 22.5242) -> (-112.7067, 22.9048)
  line L1661 (-112.7067, 22.9048) -> (-112.9306, 21.1945)
  line L1662 (-112.9306, 21.1945) -> (-112.9713, 19.4652)
  line L1663 (-112.9713, 19.4652) -> (-114.0296, 19.5975)
  line L1664 (-114.0296, 19.5975) -> (-114.8847, 20.2251)
  line L1665 (-114.8847, 20.2251) -> (-115.5886, 20.28)
  line L1666 (-115.5886, 20.28) -> (-116.1414, 19.7622)
  line L1667 (-116.1414, 19.7622) -> (-116.5431, 18.6714)
  line L1668 (-116.5431, 18.6714) -> (-116.7729, 16.6036)
  line L1669 (-116.7729, 16.6036) -> (-117.2046, 14.5704)
  line L1670 (-117.2046, 14.5704) -> (-116.8636, 13.8782)
  line L1671 (-116.8636, 13.8782) -> (-116.3971, 13.4931)
  line L1672 (-116.3971, 13.4931) -> (-115.8052, 13.4152)
  line L1673 (-115.8052, 13.4152) -> (-115.0879, 13.6444)
  line L1674 (-115.0879, 13.6444) -> (-115.3525, 11.5277)
  line L1675 (-115.3525, 11.5277) -> (-114.1747, 11.5914)
  line L1676 (-114.1747, 11.5914) -> (-113.1036, 12.0569)
  line L1677 (-113.1036, 12.0569) -> (-112.135, 14.5211)
  line L1678 (-112.135, 14.5211) -> (-111.5161, 17.0839)
  line L1679 (-111.5161, 17.0839) -> (-110.9688, 17.4923)
  line L1680 (-110.9688, 17.4923) -> (-110.61, 17.9811)
  line L1681 (-110.61, 17.9811) -> (-110.4396, 18.5506)
  line L1682 (-110.4396, 18.5506) -> (-110.4577, 19.2006)
  line L1683 (-110.4577, 19.2006) -> (-111.3216, 19.8071)
  line L1684 (-111.3216, 19.8071) -> (-111.6316, 20.4502)
  line L1685 (-111.6316, 20.4502) -> (-111.3877, 21.13)
  line L1686 (-111.3877, 21.13) -> (-110.59, 21.8464)
  line L1687 (-110.59, 21.8464) -> (-109.6324, 21.0207)
  line L1688 (-109.6324, 21.0207) -> (-108.4734, 20.5235)
  line L1689 (-108.4734, 20.5235) -> (-107.5473, 20.788)
  line L1690 (-107.5473, 20.788) -> (-106.6213, 20.5235)
  line L1691 (-106.6213, 20.5235) -> (-105.9598, 20.7881)
  line L1692 (-105.9598, 20.7881) -> (-105.7938, 21.6245)
  line L1693 (-105.7938, 21.6245) -> (-105.4307, 22.3756)
  line L1694 (-105.4307, 22.3756) -> (-104.5046, 20.3912)
  line L1695 (-104.5046, 20.3912) -> (-104.8328, 19.4115)
  line L1696 (-104.8328, 19.4115) -> (-104.9015, 18.4068)
  line L1697 (-104.9015, 18.4068) -> (-103.9753, 18.1191)
  line L1698 (-103.9753, 18.1191) -> (-103.1817, 17.6131)
  line L1699 (-103.1817, 17.6131) -> (-103.5786, 14.7027)
  line L1700 (-103.5786, 14.7027) -> (-104.2218, 13.5686)
  line L1701 (-104.2218, 13.5686) -> (-104.6369, 12.3214)
  line L1702 (-104.6369, 12.3214) -> (-104.2976, 10.5739)
  line L1703 (-104.2976, 10.5739) -> (-103.5786, 8.8819)
  line L1704 (-103.5786, 8.8819) -> (-103.2335, 9.2273)
  line L1705 (-103.2335, 9.2273) -> (-102.7848, 9.411)
  line L1706 (-102.7848, 9.411) -> (-102.1047, 9.0471)
  line L1707 (-102.1047, 9.0471) -> (-101.437, 8.9258)
  line L1708 (-101.437, 8.9258) -> (-100.7818, 9.0471)
  line L1709 (-100.7818, 9.0471) -> (-100.139, 9.411)
  line L1710 (-100.139, 9.411) -> (-98.9484, 11.9246)
  line L1711 (-98.9484, 11.9246) -> (-99.2546, 12.6812)
  line L1712 (-99.2546, 12.6812) -> (-99.3346, 13.4405)
  line L1713 (-99.3346, 13.4405) -> (-99.1884, 14.2025)
  line L1714 (-99.1884, 14.2025) -> (-98.8161, 14.9673)
  line L1715 (-98.8161, 14.9673) -> (-96.5671, 15.3641)
  line L1716 (-96.5671, 15.3641) -> (-96.3025, 16.9516)
  line L1717 (-96.3025, 16.9516) -> (-96.6949, 19.1872)
  line L1718 (-96.6949, 19.1872) -> (-97.4932, 21.3173)
  line L1719 (-97.4932, 21.3173) -> (-97.8383, 21.6627)
  line L1720 (-97.8383, 21.6627) -> (-98.2869, 21.8464)
  line L1721 (-98.2869, 21.8464) -> (-101.3296, 18.4068)
  line L1722 (-101.3296, 18.4068) -> (-102.3771, 17.9967)
  line L1723 (-102.3771, 17.9967) -> (-102.8806, 18.0805)
  line L1724 (-102.8806, 18.0805) -> (-102.8401, 18.6581)
  line L1725 (-102.8401, 18.6581) -> (-102.2557, 19.7298)
  line L1726 (-102.2557, 19.7298) -> (-98.9484, 23.9631)
  line L1727 (-98.9484, 23.9631) -> (-99.4775, 24.8891)
  line L1728 (-99.4775, 24.8891) -> (-100.3178, 24.9595)
  line L1729 (-100.3178, 24.9595) -> (-100.9948, 25.2475)
  line L1730 (-100.9948, 25.2475) -> (-101.5085, 25.7532)
  line L1731 (-101.5085, 25.7532) -> (-101.8588, 26.4766)
  line L1732 (-101.8588, 26.4766) -> (-101.6595, 27.4868)
  line L1733 (-101.6595, 27.4868) -> (-101.1962, 28.1983)
  line L1734 (-101.1962, 28.1983) -> (-100.4689, 28.6112)
  line L1735 (-100.4689, 28.6112) -> (-99.4775, 28.7256)
  line L1736 (-99.4775, 28.7256) -> (-99.3453, 29.7839)
  line L1737 (-99.3453, 29.7839) -> (-98.3749, 30.7983)
  line L1738 (-98.3749, 30.7983) -> (-97.6104, 31.9302)
  line L1739 (-97.6104, 31.9302) -> (-97.0519, 33.1796)
  line L1740 (-97.0519, 33.1796) -> (-96.6994, 34.5464)
  line L1741 (-96.6994, 34.5464) -> (-96.6734, 39.317)
  line L1742 (-96.6734, 39.317) -> (-97.0963, 44.0714)
  line L1743 (-97.0963, 44.0714) -> (-96.964, 45.1297)
  line L1744 (-96.964, 45.1297) -> (-96.3602, 46.3459)
  line L1745 (-96.3602, 46.3459) -> (-95.9164, 46.7073)
  line L1746 (-95.9164, 46.7073) -> (-95.6326, 46.2137)
  line L1747 (-95.6326, 46.2137) -> (-95.5088, 44.8651)
  line L1748 (-95.5088, 44.8651) -> (-95.9305, 42.5008)
  line L1749 (-95.9305, 42.5008) -> (-95.9057, 40.1027)
  line L1750 (-95.9057, 40.1027) -> (-95.7241, 39.5406)
  line L1751 (-95.7241, 39.5406) -> (-95.421, 39.0886)
  line L1752 (-95.421, 39.0886) -> (-94.9964, 38.7468)
  line L1753 (-94.9964, 38.7468) -> (-94.4505, 38.5152)
  line L1754 (-94.4505, 38.5152) -> (-94.2698, 37.7318)